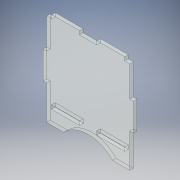
# Autodesk Inventor part: Enclosure Side
Saved by Autodesk Inventor 2018 (Build 220112000, 112)
## iProperties
Created: 2017-12-06
Part Number: Enclosure Side
Material: Glass
Document SubType Name: Modeling
Designer: Andrew
Density: 2.18 g/cm^3
Appearance: Clear
Author: Andrew
Autodesk Inventor part; units mm, degrees
ref_plane "YZ Plane" through (0, 0, 0) normal (1, 0, 0) x (0, 1, 0)
ref_plane "XZ Plane" through (0, 0, 0) normal (0, 1, 0) x (-1, 0, 0)
ref_plane "XY Plane" through (0, 0, 0) normal (0, 0, 1) x (1, 0, 0)
derived "Enclosure Top.ipt"
sketch "Sketch2" plane through (0, 0, 0) normal (0, 1, 0) x (-1, 0, 0)
  line L0 (-41.402, 93.7895) -> (-41.402, -93.7895)
  line L1 (-41.402, -93.7895) -> (41.402, -93.7895)
  line L2 (41.402, -93.7895) -> (41.402, 93.7895)
  line L3 (41.402, 93.7895) -> (-41.402, 93.7895)
  line L4 (33.576, -93.7895) -> (7.826, -93.7895)
  line L5 (7.826, -93.7895) -> (7.826, -90.4875)
  line L6 (7.826, -90.4875) -> (33.576, -90.4875)
  line L7 (33.576, -90.4875) -> (33.576, -93.7895)
  line L8 (-7.826, -93.7895) -> (-33.576, -93.7895)
  line L9 (-33.576, -93.7895) -> (-33.576, -90.4875)
  line L10 (-33.576, -90.4875) -> (-7.826, -90.4875)
  line L11 (-7.826, -90.4875) -> (-7.826, -93.7895)
  line L12 (0, -131.3053) -> (0, 131.3053)
  line L13 (-66.8528, 0) -> (66.8528, 0)
  line L14 (-41.402, -66.2073) -> (-38.1, -66.2073)
  line L15 (-38.1, -66.2073) -> (-38.1, -40.4572)
  line L16 (-38.1, -40.4572) -> (-41.402, -40.4572)
  line L17 (-41.402, -40.4572) -> (-41.402, -66.2073)
  line L18 (-41.402, -12.875) -> (-38.1, -12.875)
  line L19 (-38.1, -12.875) -> (-38.1, 12.875)
  line L20 (-38.1, 12.875) -> (-41.402, 12.875)
  line L21 (-41.402, 12.875) -> (-41.402, -12.875)
  line L22 (-41.402, 40.4572) -> (-38.1, 40.4572)
  line L23 (-38.1, 40.4572) -> (-38.1, 66.2073)
  line L24 (-38.1, 66.2073) -> (-41.402, 66.2073)
  line L25 (-41.402, 66.2073) -> (-41.402, 40.4572)
  line L26 (38.1, 50.3478) -> (36.5506, 50.3477)
  line L27 (36.5506, 50.3477) -> (36.5506, 56.3167)
  line L28 (36.5506, 56.3167) -> (38.1, 56.3167)
  line L29 (38.1, 56.3167) -> (38.1, 50.3478)
  point P0 (0, 0)
  point P1 (20.701, -90.4875)
  point P2 (-38.1, -53.3322)
  point P3 (36.5506, 53.3322)
  point P4 (-38.1, 53.3322)
derived "Enclosure Back.ipt"
sketch "Sketch2_1" plane through (0, 0, 0) normal (0, 1, 0) x (-1, 0, 0)
  line L0 (-41.402, 93.7895) -> (-41.402, -93.7895)
  line L1 (-41.402, -93.7895) -> (41.402, -93.7895)
  line L2 (41.402, -93.7895) -> (41.402, 93.7895)
  line L3 (41.402, 93.7895) -> (-41.402, 93.7895)
  line L4 (33.576, -93.7895) -> (7.826, -93.7895)
  line L5 (7.826, -93.7895) -> (7.826, -90.4875)
  line L6 (7.826, -90.4875) -> (33.576, -90.4875)
  line L7 (33.576, -90.4875) -> (33.576, -93.7895)
  line L8 (-7.826, -93.7895) -> (-33.576, -93.7895)
  line L9 (-33.576, -93.7895) -> (-33.576, -90.4875)
  line L10 (-33.576, -90.4875) -> (-7.826, -90.4875)
  line L11 (-7.826, -90.4875) -> (-7.826, -93.7895)
  line L12 (0, -131.3053) -> (0, 131.3053)
  line L13 (-66.8528, 0) -> (66.8528, 0)
  line L14 (-41.402, -66.2073) -> (-38.1, -66.2073)
  line L15 (-38.1, -66.2073) -> (-38.1, -40.4572)
  line L16 (-38.1, -40.4572) -> (-41.402, -40.4572)
  line L17 (-41.402, -40.4572) -> (-41.402, -66.2073)
  line L18 (-41.402, -12.875) -> (-38.1, -12.875)
  line L19 (-38.1, -12.875) -> (-38.1, 12.875)
  line L20 (-38.1, 12.875) -> (-41.402, 12.875)
  line L21 (-41.402, 12.875) -> (-41.402, -12.875)
  line L22 (-41.402, 40.4572) -> (-38.1, 40.4572)
  line L23 (-38.1, 40.4572) -> (-38.1, 66.2073)
  line L24 (-38.1, 66.2073) -> (-41.402, 66.2073)
  line L25 (-41.402, 66.2073) -> (-41.402, 40.4572)
  line L26 (38.1, 50.3478) -> (36.5506, 50.3477)
  line L27 (36.5506, 50.3477) -> (36.5506, 56.3167)
  line L28 (36.5506, 56.3167) -> (38.1, 56.3167)
  line L29 (38.1, 56.3167) -> (38.1, 50.3478)
  point P0 (0, 0)
  point P1 (20.701, -90.4875)
  point P2 (-38.1, -53.3322)
  point P3 (36.5506, 53.3322)
  point P4 (-38.1, 53.3322)
sketch "Sketch3" plane through (0, 0, 0) normal (1, 0, 0) x (0, 1, 0)
  line L0 (0, 93.7895) -> (0, -93.7895)
  line L1 (0, 93.7895) -> (-87.817, 93.7895)
  line L2 (-87.817, -93.7895) -> (0, -93.7895)
  line L3 (-3.302, 93.7895) -> (-3.302, -93.7895) construction
  line L4 (-71.592, 93.7895) -> (-71.592, -93.7895) construction
  line L5 (-75.117, 93.7895) -> (-75.117, -93.7895) construction
  line L6 (-87.817, 93.7895) -> (-87.817, 74.7395)
  line L7 (-87.817, -93.7895) -> (-87.817, -74.7395)
  arc A0 (-87.817, -74.7395) -> (-87.817, 74.7395) centre (-376.2825, 0) ccw
  line L8 (-71.592, 66.2073) -> (-75.117, 66.2073)
  line L9 (-75.117, 66.2073) -> (-75.117, 40.4573)
  line L10 (-75.117, 40.4573) -> (-71.592, 40.4573)
  line L11 (-71.592, 40.4573) -> (-71.592, 66.2073)
  line L12 (-71.592, 12.875) -> (-75.117, 12.875)
  line L13 (-75.117, 12.875) -> (-75.117, -12.875)
  line L14 (-75.117, -12.875) -> (-71.592, -12.875)
  line L15 (-71.592, -12.875) -> (-71.592, 12.875)
  line L16 (-71.592, -40.4573) -> (-75.117, -40.4573)
  line L17 (-75.117, -40.4573) -> (-75.117, -66.2073)
  line L18 (-75.117, -66.2073) -> (-71.592, -66.2073)
  line L19 (-71.592, -66.2073) -> (-71.592, -40.4573)
  line L20 (-451.5389, 0) -> (75.2565, 0)
  circle A1 centre (-4.826, 53.3322) radius 1.4605
  point P0 (0, 0)
  point P1 (0, -53.3322)
  point P2 (-71.592, -53.3323)
sketch "Sketch4" plane through (0, 0, 0) normal (1, 0, 0) x (0, 1, 0)
  line L0 (-451.5389, 0) -> (75.2565, 0)
  line L1 (0, 93.7895) -> (-87.817, 93.7895)
  line L2 (-87.817, -93.7895) -> (0, -93.7895)
  line L3 (0, 93.7895) -> (0, -93.7895)
  line L4 (0, -40.6323) -> (-3.302, -40.6323)
  line L5 (-3.302, -40.6323) -> (-3.302, -12.7)
  line L6 (-3.302, -12.7) -> (0, -12.7)
  line L7 (0, -12.7) -> (0, -40.6323)
  line L8 (0, -66.0323) -> (-3.302, -66.0323)
  line L9 (-3.302, -66.0323) -> (-3.302, -93.7895)
  line L10 (-3.302, -93.7895) -> (0, -93.7895)
  line L11 (0, -93.7895) -> (0, -66.0323)
  line L12 (0, 12.7) -> (-3.302, 12.7)
  line L13 (-3.302, 12.7) -> (-3.302, 40.6323)
  line L14 (-3.302, 40.6323) -> (0, 40.6323)
  line L15 (0, 40.6323) -> (0, 12.7)
  line L16 (0, 66.0323) -> (-3.302, 66.0323)
  line L17 (-3.302, 66.0323) -> (-3.302, 93.7895)
  line L18 (-3.302, 93.7895) -> (0, 93.7895)
  line L19 (0, 93.7895) -> (0, 66.0323)
  line L20 (-87.817, -93.7895) -> (-87.817, -74.7395)
  arc A0 (-87.817, -74.7395) -> (-87.817, 74.7395) centre (-376.2825, 0) ccw
  line L21 (-87.817, 93.7895) -> (-87.817, 74.7395)
  line L22 (-31.0335, 93.7895) -> (-56.7835, 93.7895)
  line L23 (-56.7835, 93.7895) -> (-56.7835, 90.4875)
  line L24 (-56.7835, 90.4875) -> (-31.0335, 90.4875)
  line L25 (-31.0335, 90.4875) -> (-31.0335, 93.7895)
  line L26 (-71.592, 93.7895) -> (-71.592, -93.7895) construction
  line L27 (-75.117, 93.7895) -> (-75.117, -93.7895) construction
  line L28 (-31.0335, -93.7895) -> (-56.7835, -93.7895)
  line L29 (-56.7835, -93.7895) -> (-56.7835, -90.4875)
  line L30 (-56.7835, -90.4875) -> (-31.0335, -90.4875)
  line L31 (-31.0335, -90.4875) -> (-31.0335, -93.7895)
  point P0 (0, 0)
  point P1 (0, -53.3322)
  point P2 (-43.9085, 90.4875)
  point P3 (-43.9085, 93.7895)
sketch "Sketch6" plane through (0, 0, 0) normal (0, 0, 1) x (1, 0, 0)
  line L0 (0, 0) -> (0, -87.817) construction
  line L1 (41.402, 0) -> (-41.402, 0) projected
  line L2 (-41.402, 0) -> (-41.402, -87.817)
  line L3 (-41.402, -87.817) -> (-22.352, -87.817)
  line L4 (41.402, 0) -> (41.402, -87.817)
  line L5 (41.402, -87.817) -> (22.352, -87.817)
  arc A0 (22.352, -87.817) -> (-22.352, -87.817) centre (0, -109.2808) ccw
  line L6 (-41.402, -75.117) -> (41.402, -75.117) construction
  line L7 (41.402, -71.592) -> (-41.402, -71.592) construction
  line L8 (-33.576, -71.592) -> (-7.826, -71.592)
  line L9 (-7.826, -71.592) -> (-7.826, -75.117)
  line L10 (-7.826, -75.117) -> (-33.576, -75.117)
  line L11 (-33.576, -75.117) -> (-33.576, -71.592)
  line L12 (7.826, -71.592) -> (33.576, -71.592)
  line L13 (33.576, -71.592) -> (33.576, -75.117)
  line L14 (33.576, -75.117) -> (7.826, -75.117)
  line L15 (7.826, -75.117) -> (7.826, -71.592)
  line L16 (-20.701, -71.592) -> (-20.701, -75.117) construction
  point P0 (0, -71.592)
  point P1 (0, -75.117)
  dimension "d2" = 19.05
  dimension "d3" = 3.175
  dimension "d12" = 25.75
  dimension "d13" = 20.701
  dimension "d14" = 41.402
  constraints: 30 end point, 9 point on line, 6 perpendicular, 4 midpoint, 4 parallel, 3 collinear, 2 horizontal, 2 point on circle, 2 vertical, 1 centre point, 1 other
  measures "d2" distance of L2.end L3.end
  measures "d3" distance edge to line of A0 L6
  measures "d12" distance of L8.start L8.end
  measures "d13" distance between parallel lines of L0 L16
  measures "d14" distance between parallel lines of L2 L0
extrude "Extrusion1" add sketch "Sketch6" along normal blind 3.302
sketch "Sketch7" plane through (0, 0, 0) normal (0, 0, 1) x (1, 0, 0)
  line L0 (-41.402, 0) -> (-41.402, -87.817) projected
  line L1 (-41.402, -87.817) -> (-22.352, -87.817) projected
  arc A0 (22.352, -87.817) -> (-22.352, -87.817) centre (0, -109.2808) ccw projected
  line L2 (41.402, -87.817) -> (22.352, -87.817) projected
  line L3 (41.402, 0) -> (41.402, -87.817) projected
  line L4 (41.402, 0) -> (-41.402, 0) projected
  line L5 (-41.402, 0) -> (-33.401, 0)
  line L6 (-33.401, 0) -> (-33.401, -3.302)
  line L7 (-33.401, -3.302) -> (-41.402, -3.302)
  line L8 (-41.402, -3.302) -> (-41.402, 0)
  line L9 (33.401, 0) -> (41.402, 0)
  line L10 (41.402, 0) -> (41.402, -3.302)
  line L11 (41.402, -3.302) -> (33.401, -3.302)
  line L12 (33.401, -3.302) -> (33.401, 0)
  line L13 (-8.001, 0) -> (8.001, 0)
  line L14 (8.001, 0) -> (8.001, -3.302)
  line L15 (8.001, -3.302) -> (-8.001, -3.302)
  line L16 (-8.001, -3.302) -> (-8.001, 0)
  line L17 (0, 75.2565) -> (0, -451.5389) projected
  line L18 (41.402, -3.302) -> (38.1, -3.302)
  line L19 (38.1, -3.302) -> (38.1, -31.2085)
  line L20 (38.1, -31.2085) -> (41.402, -31.2085)
  line L21 (41.402, -31.2085) -> (41.402, -3.302)
  line L22 (-41.402, -3.302) -> (-38.1, -3.302)
  line L23 (-38.1, -3.302) -> (-38.1, -31.2085)
  line L24 (-38.1, -31.2085) -> (-41.402, -31.2085)
  line L25 (-41.402, -31.2085) -> (-41.402, -3.302)
  line L26 (-41.402, -87.817) -> (-38.1, -87.817)
  line L27 (-38.1, -87.817) -> (-38.1, -56.6085)
  line L28 (-38.1, -56.6085) -> (-41.402, -56.6085)
  line L29 (-41.402, -56.6085) -> (-41.402, -87.817)
  line L30 (41.402, -87.817) -> (38.1, -87.817)
  line L31 (38.1, -87.817) -> (38.1, -56.6085)
  line L32 (38.1, -56.6085) -> (41.402, -56.6085)
  line L33 (41.402, -56.6085) -> (41.402, -87.817)
  line L34 (38.1, -31.2085) -> (38.1, -56.6085) construction
  point P0 (0, 0)
  point P1 (-20.701, 0)
  point P2 (38.1, -43.9085)
  point P3 (41.402, -43.9085)
  dimension "d6" = 3.302
  dimension "d7" = 25.4
  dimension "d8" = 12.7
  dimension "d9" = 25.4
  constraints: 58 end point, 14 parallel, 9 perpendicular, 7 horizontal, 6 point on line, 5 collinear, 2 midpoint, 1 horizontal alignment, 1 vertical, 2 other
  measures "d6" distance of L5.end L6.end
  measures "d7" distance between parallel lines of L6 L16
  measures "d8" distance from line of L16 point (-20.701, 0)
  measures "d9" distance between parallel lines of L32 L20
extrude "Extrusion2" cut sketch "Sketch7" along normal blind 3.302 contours L4 L6 L7 L0 | L7 L23 L24 L0 | L4 L17 L15 L16 | L28 L27 L1 L0 | L4 L14 L15 L17 | L4 L3 L11 L12 | L3 L20 L19 L11 | L31 L32 L3 L2
equation "\"d13\" = 0.5 * d14"
equation "\"d4\" = encThick"
equation "\"d6\" = encThick"
equation "\"d7\" = encTab"
equation "\"d8\" = 0.5 * d7"
equation "\"d9\" = encTab"
equation "\"d10\" = encThick"
equation "\"encThick\" = 3.302"
equation "\"encTab\" = 25.4"
body "Solid1"
